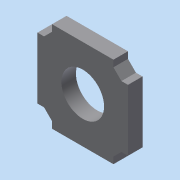
# Autodesk Inventor part: 20_Cube_Insert_Holder-okular+flashlight_v3
Saved by Autodesk Inventor 2019.4 (Build 234330000, 330)
## iProperties
Created: 2019-07-24
Part Number: 20_Cube_Insert_Holder-okular+flashlight_v3
Material: Generic
Document SubType Name: Modeling
Designer: marsikovabarbora
Density: 1 g/cm^3
Appearance: Default
Author: marsikovabarbora
Autodesk Inventor part; units mm, degrees
ref_plane "YZ Plane" through (0, 0, 0) normal (1, 0, 0) x (0, 1, 0)
ref_plane "XZ Plane" through (0, 0, 0) normal (0, 1, 0) x (-1, 0, 0)
ref_plane "XY Plane" through (0, 0, 0) normal (0, 0, 1) x (1, 0, 0)
sketch "Sketch1" plane through (0, 0, 0) normal (0, 0, 1) x (1, 0, 0)
  line L0 (21.5871, 13.6345) -> (17.0871, 18.1345) projected
  line L1 (17.0871, 18.1345) -> (-16.7129, 18.1345) projected
  line L2 (-16.7129, 18.1345) -> (-21.2129, 13.6345) projected
  line L3 (-21.0966, 13.6345) -> (-21.0966, -20.1655) projected
  line L4 (21.4709, -20.1655) -> (21.4709, 13.6345) projected
  line L5 (21.4709, -20.1655) -> (17.0871, -24.4078) projected
  line L6 (-16.7129, -24.4078) -> (17.0871, -24.4078) projected
  line L7 (-16.7129, -24.4078) -> (-21.0966, -20.1655) projected
  line L8 (-24.7129, -28.1655) -> (-24.7129, 13.6345) construction
  line L9 (25.0871, -28.1655) -> (-24.7129, -28.1655) construction
  line L10 (25.0871, -28.1655) -> (25.0871, 13.6345) construction
  line L11 (17.0871, 21.6345) -> (-16.7129, 21.6345) construction
  line L12 (0.1871, -36.5255) -> (0.1871, 21.9945)
  line L13 (14.6206, -3.2655) -> (-14.2825, -3.2655) construction
  line L14 (-21.0552, -20.0655) -> (-16.6129, -24.5078)
  line L15 (-16.6129, -24.5078) -> (-16.6129, -28.1655)
  line L16 (-16.6129, -28.1655) -> (16.9871, -28.1655)
  line L17 (16.9871, -28.1655) -> (16.9871, -24.5078)
  line L18 (16.9871, -24.5078) -> (21.4295, -20.0655)
  line L19 (25.0871, -20.0655) -> (21.4295, -20.0655)
  line L20 (25.0871, 13.5345) -> (25.0871, -20.0655)
  line L21 (21.4295, 13.5345) -> (25.0871, 13.5345)
  line L22 (21.4295, 13.5345) -> (16.9871, 17.9768)
  line L23 (16.9871, 17.9768) -> (16.9871, 21.6345)
  line L24 (16.9871, 21.6345) -> (-16.6129, 21.6345)
  line L25 (-16.6129, 21.6345) -> (-16.6129, 17.9768)
  line L26 (-16.6129, 17.9768) -> (-21.0552, 13.5345)
  line L27 (-24.7129, 13.5345) -> (-21.0552, 13.5345)
  line L28 (-24.7129, -20.0655) -> (-24.7129, 13.5345)
  line L29 (-21.0552, -20.0655) -> (-24.7129, -20.0655)
  circle A0 centre (0.1871, -3.2655) radius 11.75
  point P0 (14.2, -44.8454)
  point P1 (11.9334, -2.9712)
  point P2 (-1.4501, -14.9009)
  point P3 (-5.6, -13.4915)
  point P4 (-9.0465, 4.0011)
  point P5 (-6.23, 6.5774)
  point P6 (11.3484, 0.4071)
  point P7 (16.9871, 19.8057)
  dimension "d48" = 23.5
  constraints: 36 end point, 8 horizontal, 6 point on circle, 6 vertical, 1 centre point, 1 midpoint, 7 other
  measures "d48" diameter of A0
extrude "Extrusion1" add sketch "Sketch1" along normal blind 8 contours L23 L22 L21 L4 L19 L18 L6 L12 A0 L1 | L1 L12 L24 L23 | L12 A0 L6 L14 L29 L3 L27 L26 L25 L1 | L1 L25 L24 L12 | L21 L20 L19 L4 | L12 L16 L15 L14 L6 | L6 L18 L17 L16 L12 | L3 L29 L28 L27
sketch "Skizze3" plane through (0, 0, 8) normal (0, 0, 1) x (1, 0, 0)
  circle A0 centre (0.1871, -3.2655) radius 11.75 construction
  line L0 (-21.0552, -20.0655) -> (-16.6129, -24.5078) projected
  line L1 (-16.6129, -24.5078) -> (-16.6129, -28.1655) projected
  line L2 (-16.6129, -28.1655) -> (16.9871, -28.1655) construction
  line L3 (16.9871, -28.1655) -> (16.9871, -24.5078) projected
  line L4 (16.9871, -24.5078) -> (21.4295, -20.0655) projected
  line L5 (21.4295, -20.0655) -> (25.0871, -20.0655) projected
  line L6 (25.0871, -20.0655) -> (25.0871, 13.5345) construction
  line L7 (25.0871, 13.5345) -> (21.4295, 13.5345) projected
  line L8 (21.4295, 13.5345) -> (16.9871, 17.9768) projected
  line L9 (16.9871, 17.9768) -> (16.9871, 21.6345) projected
  line L10 (16.9871, 21.6345) -> (-16.6129, 21.6345) construction
  line L11 (-16.6129, 21.6345) -> (-16.6129, 17.9768) projected
  line L12 (-16.6129, 17.9768) -> (-21.0552, 13.5345) projected
  line L13 (-21.0552, 13.5345) -> (-24.7129, 13.5345) projected
  line L14 (-24.7129, 13.5345) -> (-24.7129, -20.0655) construction
  line L15 (-24.7129, -20.0655) -> (-21.0552, -20.0655) projected
  line L16 (-16.7129, 21.7345) -> (17.0871, 21.7345) construction
  line L17 (17.0871, 21.7345) -> (17.0871, 18.0183)
  line L18 (17.0871, 18.0183) -> (21.4709, 13.6345)
  line L19 (21.4709, 13.6345) -> (25.1871, 13.6345)
  line L20 (25.1871, 13.6345) -> (25.1871, -20.1655) construction
  line L21 (25.1871, -20.1655) -> (21.4709, -20.1655)
  line L22 (21.4709, -20.1655) -> (17.0871, -24.5493)
  line L23 (17.0871, -24.5493) -> (17.0871, -28.2655)
  line L24 (17.0871, -28.2655) -> (-16.7129, -28.2655) construction
  line L25 (-16.7129, -28.2655) -> (-16.7129, -24.5493)
  line L26 (-16.7129, -24.5493) -> (-21.0966, -20.1655)
  line L27 (-21.0966, -20.1655) -> (-24.8129, -20.1655)
  line L28 (-24.8129, -20.1655) -> (-24.8129, 13.6345) construction
  line L29 (-24.8129, 13.6345) -> (-21.0966, 13.6345)
  line L30 (-21.0966, 13.6345) -> (-16.7129, 18.0183)
  line L31 (-16.7129, 18.0183) -> (-16.7129, 21.7345)
  line L32 (-21.0552, 13.5345) -> (-24.7129, 13.5345) projected
  line L33 (-24.7129, 13.5345) -> (-24.7129, 13.6345)
  line L34 (-16.6129, 21.6345) -> (-16.7129, 21.6345)
  line L35 (16.9871, 21.6345) -> (17.0871, 21.6345)
  line L36 (25.0871, 13.5345) -> (25.0871, 13.6345)
  line L37 (25.0871, -20.0655) -> (25.0871, -20.1655)
  line L38 (-16.6129, -28.1655) -> (16.9871, -28.1655) projected
  line L39 (16.9871, -28.1655) -> (17.0871, -28.1655)
  line L40 (-16.6129, -28.1655) -> (-16.7129, -28.1655)
  line L41 (-24.7129, -20.0655) -> (-24.7129, -20.1655)
  point P0 (0, 0)
  dimension "d52" = 0.1
  constraints: 48 end point, 12 point on line, 3 perpendicular, 1 collinear, 15 other
  measures "d52" distance between parallel lines of L10 L16
extrude "IM_offset" add sketch "Skizze3" against normal up to surface (8 mm away)
body "Solid1"
